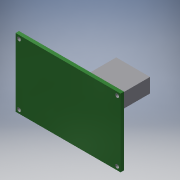
# Autodesk Inventor part: PCB
Saved by Autodesk Inventor 2018 (Build 220112000, 112)
## iProperties
Created: 2018-05-21
Part Number: PCB
Material: Generic
Document SubType Name: Modeling
Designer: David
Density: 1 g/cm^3
Appearance: Default
Author: David
Autodesk Inventor part; units mm, degrees
ref_plane "YZ Plane" through (0, 0, 0) normal (1, 0, 0) x (0, 1, 0)
ref_plane "XZ Plane" through (0, 0, 0) normal (0, 1, 0) x (-1, 0, 0)
ref_plane "XY Plane" through (0, 0, 0) normal (0, 0, 1) x (1, 0, 0)
sketch "Sketch1" plane through (0, 0, 0) normal (0, 1, 0) x (-1, 0, 0)
  line L0 (-45.5, -29.5) -> (45.5, -29.5)
  line L1 (45.5, -29.5) -> (45.5, 29.5)
  line L2 (45.5, 29.5) -> (-45.5, 29.5)
  line L3 (-45.5, 29.5) -> (-45.5, -29.5)
  line L4 (-45.5, -29.5) -> (45.5, 29.5) construction
  line L5 (45.5, -29.5) -> (-45.5, 29.5) construction
  point P0 (0, 0)
  dimension "d0" = 91
  dimension "d1" = 59
  constraints: 12 end point, 2 midpoint, 2 parallel, 1 horizontal, 1 perpendicular
  measures "d0" distance of L2.end L1.end
  measures "d1" distance of L1.end L0.end
extrude "Extrusion1" add sketch "Sketch1" along normal blind 3
sketch "Sketch2" plane through (0, 3, 0) normal (0, 1, 0) x (1, 0, 0)
  line L0 (45.5, 29.5) -> (-45.5, 29.5) projected
  line L1 (-45.5, 29.5) -> (-43, 29.5)
  line L2 (-43, 29.5) -> (-43, 22.5)
  line L3 (-43, 22.5) -> (-45.5, 22.5)
  line L4 (-45.5, 22.5) -> (-45.5, 29.5)
  line L5 (-43, 22.5) -> (5, 22.5)
  line L6 (5, 22.5) -> (5, 2.1)
  line L7 (5, 2.1) -> (-43, 2.1)
  line L8 (-43, 2.1) -> (-43, 22.5)
  line L9 (6.7, 19.2) -> (28.8, 19.2)
  line L10 (28.8, 19.2) -> (28.8, 3.9)
  line L11 (28.8, 3.9) -> (6.7, 3.9)
  line L12 (6.7, 3.9) -> (6.7, 19.2)
  line L13 (6.7, 19.2) -> (28.8, 3.9) construction
  line L14 (28.8, 19.2) -> (6.7, 3.9) construction
  line L15 (3.7, -4.4) -> (33, -4.4)
  line L16 (33, -4.4) -> (33, -16.8)
  line L17 (33, -16.8) -> (3.7, -16.8)
  line L18 (3.7, -16.8) -> (3.7, -4.4)
  line L19 (3.7, -4.4) -> (33, -16.8) construction
  line L20 (33, -4.4) -> (3.7, -16.8) construction
  line L21 (45.5, -29.5) -> (45.5, 29.5) projected
  line L22 (-45.5, -29.5) -> (45.5, -29.5) projected
  point P0 (0, 0)
  point P1 (17.75, 11.55)
  point P2 (18.35, -10.6)
  dimension "d4" = 2.5
  dimension "d5" = 7
  dimension "d6" = 48
  dimension "d7" = 20.4
  dimension "d10" = 1.7
  dimension "d11" = 22.1
  dimension "d12" = 15.3
  dimension "d13" = 3.3
  dimension "d14" = 12.4
  dimension "d15" = 29.3
  dimension "d16" = 12.5
  dimension "d17" = 12.7
  constraints: 40 end point, 8 parallel, 4 horizontal, 4 midpoint, 4 perpendicular
  measures "d4" distance of L2.end L3.end
  measures "d5" distance of L1.end L2.end
  measures "d6" distance of L6.end L7.end
  measures "d7" distance of L5.end L6.end
  measures "d10" distance between parallel lines of L12 L6
  measures "d11" distance of L10.end L11.end
  measures "d12" distance of L9.end L10.end
  measures "d13" distance between parallel lines of L5 L9
  measures "d14" distance of L15.end L16.end
  measures "d15" distance of L16.end L17.end
  measures "d16" distance between parallel lines of L21 L16
  measures "d17" distance between parallel lines of L22 L17
extrude "Extrusion2" add sketch "Sketch2" along normal blind 10 contours L5 L6 L7 L8 | L9 L10 L11 L12 | L15 L16 L17 L18
sketch "Sketch3" plane through (0, 3, 0) normal (0, 1, 0) x (1, 0, 0)
  line L0 (-42.5, 26.5) -> (42.5, 26.5)
  line L1 (42.5, 26.5) -> (42.5, -26.5)
  line L2 (42.5, -26.5) -> (-42.5, -26.5)
  line L3 (-42.5, -26.5) -> (-42.5, 26.5)
  line L4 (-42.5, 26.5) -> (42.5, -26.5) construction
  line L5 (42.5, 26.5) -> (-42.5, -26.5) construction
  circle A0 centre (42.5, -26.5) radius 1.6
  circle A1 centre (-42.5, -26.5) radius 1.6
  circle A2 centre (-42.5, 26.5) radius 1.6
  circle A3 centre (42.5, 26.5) radius 1.6
  point P0 (0, 0)
  dimension "d18" = 85
  dimension "d19" = 53
  dimension "d20" = 3.2
  dimension "d21" = 3.2
  dimension "d22" = 3.2
  dimension "d23" = 3.2
  constraints: 12 end point, 4 centre point, 4 coincident, 2 midpoint, 2 parallel, 1 horizontal, 1 perpendicular
  measures "d18" distance of L1.end L2.end
  measures "d19" distance of L0.end L1.end
  measures "d20" diameter of A0
  measures "d21" diameter of A1
  measures "d22" diameter of A2
  measures "d23" diameter of A3
extrude "Extrusion3" cut sketch "Sketch3" against normal blind 3 contours L3 A2 L0 | L0 A2 L3 | A3 L1 L0 | L0 L1 A3 | A1 L2 L3 | L3 L2 A1 | A0 L2 L1 | L1 L2 A0
sketch "Sketch4" plane through (0, 13, 0) normal (0, 1, 0) x (1, 0, 0)
  line L0 (3.7, -4.4) -> (3.7, -16.8) projected
  line L1 (3.7, -4.4) -> (33, -4.4) projected
  line L2 (3.7, -16.8) -> (33, -16.8)
  line L3 (33, -16.8) -> (33, -4.4)
  line L4 (33, -4.4) -> (3.7, -4.4)
  line L5 (3.7, -4.4) -> (3.7, -16.8)
  point P0 (0, 0)
  constraints: 8 end point, 2 parallel, 1 horizontal, 1 perpendicular
extrude "Extrusion4" add sketch "Sketch4" along normal blind 25
body "Solid1"
